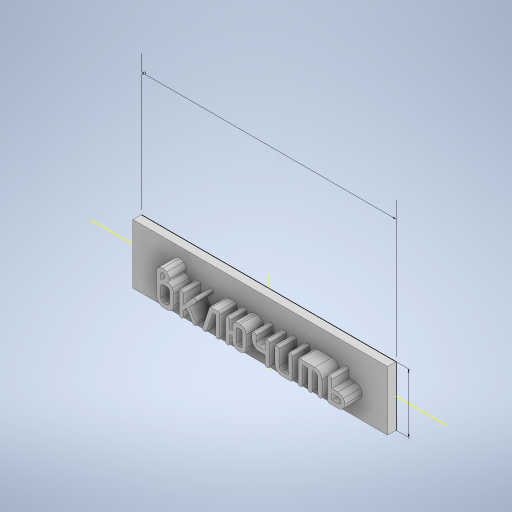
# Autodesk Inventor part: test hard text
Saved by Autodesk Inventor 2023.1 (Build 271208000, 208)
## iProperties
Created: 2023-03-05
Part Number: test hard text
Material: Типовые
Document SubType Name: Modeling
Designer: User
Density: 1 g/cm^3
Appearance: По умолчанию
Author: User
Autodesk Inventor part; units mm, degrees
ref_plane "YZ Plane" through (0, 0, 0) normal (1, 0, 0) x (0, 1, 0)
ref_plane "XZ Plane" through (0, 0, 0) normal (0, 1, 0) x (-1, 0, 0)
ref_plane "XY Plane" through (0, 0, 0) normal (0, 0, 1) x (1, 0, 0)
sketch "Эскиз1" plane through (0, 0, 0) normal (0, 0, 1) x (1, 0, 0)
  line L0 (-15, 3.5) -> (15, 3.5)
  line L1 (15, 3.5) -> (15, -3.5)
  line L2 (15, -3.5) -> (-15, -3.5)
  line L3 (-15, -3.5) -> (-15, 3.5)
  line L4 (0, -4.9) -> (0, 4.9) projected
  line L5 (-21, 0) -> (21, 0) projected
  line L6 (-10.6132, 2.2995) -> (12.268, 2.2995) construction
  line L7 (12.268, 2.2995) -> (12.268, -1.6939) construction
  line L8 (12.268, -1.6939) -> (-10.6132, -1.6939) construction
  line L9 (-10.6132, -1.6939) -> (-10.6132, 2.2995) construction
  spline S0 degree 2 poles (-8.9465, 1.1246) (-8.6066, 1.1246) (-8.3624, 0.8441) knots 0 0 0 1 1 1
  spline S1 degree 2 poles (-8.3624, 0.8441) (-8.1743, 0.6626) (-8.1743, 0.3061) knots 0 0 0 1 1 1
  line L10 (-8.1743, 0.3061) -> (-8.1743, -0.8556)
  spline S2 degree 2 poles (-8.1743, -0.8556) (-8.1743, -1.1988) (-8.6594, -1.6873) (-9.0059, -1.6873) knots 0 0 0 1 2 2 2
  line L11 (-9.0059, -1.6873) -> (-9.3954, -1.6873)
  spline S3 degree 2 poles (-9.3954, -1.6873) (-9.7353, -1.6873) (-10.2238, -1.2021) (-10.2238, -0.8556) knots 0 0 0 1 2 2 2
  line L12 (-10.2238, -0.8556) -> (-10.2238, 1.5471)
  spline S4 degree 2 poles (-10.2238, 1.5471) (-10.2238, 1.9002) (-9.9894, 2.1114) knots 0 0 0 1 1 1
  spline S5 degree 2 poles (-9.9894, 2.1114) (-9.7749, 2.2995) (-9.468, 2.2995) knots 0 0 0 1 1 1
  spline S6 degree 2 poles (-9.468, 2.2995) (-9.1611, 2.2995) (-9.0191, 2.1279) knots 0 0 0 1 1 1
  spline S7 degree 2 poles (-9.0191, 2.1279) (-8.7155, 1.9035) (-8.7155, 1.5504) knots 0 0 0 1 1 1
  spline S8 degree 2 poles (-8.7155, 1.5504) (-8.7155, 1.1939) (-8.9465, 1.1246) knots 0 0 0 1 1 1
  line L13 (-8.6759, -0.8589) -> (-8.6759, 0.3061)
  spline S9 degree 2 poles (-8.6759, 0.3061) (-8.6759, 0.4381) (-8.8739, 0.6362) (-9.0059, 0.6362) knots 0 0 0 1 2 2 2
  line L14 (-9.0059, 0.6362) -> (-9.3954, 0.6362)
  spline S10 degree 2 poles (-9.3954, 0.6362) (-9.5274, 0.6362) (-9.7221, 0.4414) (-9.7221, 0.3061) knots 0 0 0 1 2 2 2
  line L15 (-9.7221, 0.3061) -> (-9.7221, -0.8589)
  spline S11 degree 2 poles (-9.7221, -0.8589) (-9.7221, -0.9942) (-9.5274, -1.1889) (-9.3954, -1.1889) knots 0 0 0 1 2 2 2
  line L16 (-9.3954, -1.1889) -> (-9.0059, -1.1889)
  spline S12 degree 2 poles (-9.0059, -1.1889) (-8.8706, -1.1889) (-8.6759, -0.9942) (-8.6759, -0.8589) knots 0 0 0 1 2 2 2
  spline S13 degree 2 poles (-9.7221, 1.0025) (-9.6627, 1.0883) (-9.435, 1.2533) knots 0 0 0 1 1 1
  spline S14 degree 2 poles (-9.435, 1.2533) (-9.2172, 1.4249) (-9.2172, 1.5438) knots 0 0 0 1 1 1
  spline S15 degree 2 poles (-9.2172, 1.5438) (-9.2172, 1.6659) (-9.3063, 1.7451) knots 0 0 0 1 1 1
  spline S16 degree 2 poles (-9.3063, 1.7451) (-9.369, 1.7946) (-9.4713, 1.7946) knots 0 0 0 1 1 1
  spline S17 degree 2 poles (-9.4713, 1.7946) (-9.5769, 1.7946) (-9.6264, 1.7781) knots 0 0 0 1 1 1
  spline S18 degree 2 poles (-9.6264, 1.7781) (-9.7221, 1.6659) (-9.7221, 1.5438) knots 0 0 0 1 1 1
  line L17 (-9.7221, 1.5438) -> (-9.7221, 1.0025)
  spline S19 degree 2 poles (-6.6825, -0.4199) (-6.732, -0.4595) (-7.0489, -0.8391) knots 0 0 0 1 1 1
  line L18 (-7.0489, -0.8391) -> (-7.0489, -1.4364)
  spline S20 degree 2 poles (-7.0489, -1.4364) (-7.0489, -1.6873) (-7.2997, -1.6873) knots 0 0 0 1 1 1
  spline S21 degree 2 poles (-7.2997, -1.6873) (-7.5505, -1.6873) (-7.5505, -1.4364) knots 0 0 0 1 1 1
  line L19 (-7.5505, -1.4364) -> (-7.5505, 0.887)
  spline S22 degree 2 poles (-7.5505, 0.887) (-7.5505, 1.1378) (-7.2997, 1.1378) knots 0 0 0 1 1 1
  spline S23 degree 2 poles (-7.2997, 1.1378) (-7.0489, 1.1378) (-7.0489, 0.887) knots 0 0 0 1 1 1
  line L20 (-7.0489, 0.887) -> (-7.0489, -0.1988)
  line L21 (-7.0489, -0.1988) -> (-5.8805, 1.0883)
  spline S24 degree 2 poles (-5.8805, 1.0883) (-5.8508, 1.1477) (-5.7551, 1.1477) knots 0 0 0 1 1 1
  spline S25 degree 2 poles (-5.7551, 1.1477) (-5.6528, 1.1477) (-5.5043, 0.9827) (-5.5043, 0.8837) knots 0 0 0 1 2 2 2
  spline S26 degree 2 poles (-5.5043, 0.8837) (-5.5043, 0.7781) (-5.5802, 0.7022) knots 0 0 0 1 1 1
  line L22 (-5.5802, 0.7022) -> (-6.3426, -0.0833)
  line L23 (-6.3426, -0.0833) -> (-5.5604, -1.2747)
  spline S27 degree 2 poles (-5.5604, -1.2747) (-5.5043, -1.3605) (-5.5043, -1.4397) knots 0 0 0 1 1 1
  spline S28 degree 2 poles (-5.5043, -1.4397) (-5.5043, -1.5454) (-5.6627, -1.6939) (-5.7584, -1.6939) knots 0 0 0 1 2 2 2
  spline S29 degree 2 poles (-5.7584, -1.6939) (-5.8805, -1.6939) (-5.9168, -1.618) knots 0 0 0 1 1 1
  line L24 (-5.9168, -1.618) -> (-6.6825, -0.4199)
  spline S30 degree 2 poles (-2.7452, -1.4364) (-2.7452, -1.6873) (-2.996, -1.6873) knots 0 0 0 1 1 1
  spline S31 degree 2 poles (-2.996, -1.6873) (-3.2469, -1.6873) (-3.2469, -1.4364) knots 0 0 0 1 1 1
  line L25 (-3.2469, -1.4364) -> (-3.2469, 0.6395)
  line L26 (-3.2469, 0.6395) -> (-3.5934, 0.6395)
  line L27 (-3.5934, 0.6395) -> (-4.3195, -1.5553)
  spline S32 degree 2 poles (-4.3195, -1.5553) (-4.3591, -1.6873) (-4.534, -1.6873) knots 0 0 0 1 1 1
  spline S33 degree 2 poles (-4.534, -1.6873) (-4.7914, -1.6873) (-4.7914, -1.4463) knots 0 0 0 1 1 1
  spline S34 degree 2 poles (-4.7914, -1.4463) (-4.7914, -1.4001) (-4.7782, -1.3572) knots 0 0 0 1 1 1
  line L28 (-4.7782, -1.3572) -> (-3.996, 1.0058)
  spline S35 degree 2 poles (-3.996, 1.0058) (-3.9564, 1.1378) (-3.7749, 1.1378) knots 0 0 0 1 1 1
  line L29 (-3.7749, 1.1378) -> (-2.996, 1.1378)
  spline S36 degree 2 poles (-2.996, 1.1378) (-2.7452, 1.1378) (-2.7452, 0.887) knots 0 0 0 1 1 1
  line L30 (-2.7452, 0.887) -> (-2.7452, -1.4364)
  line L31 (-1.5769, -0.0272) -> (-1.3063, -0.0272)
  line L32 (-1.3063, -0.0272) -> (-1.3063, 0.4216)
  spline S37 degree 2 poles (-1.3063, 0.4216) (-1.3063, 0.7154) (-0.8904, 1.1378) (-0.5901, 1.1378) knots 0 0 0 1 2 2 2
  line L33 (-0.5901, 1.1378) -> (-0.3591, 1.1378)
  spline S38 degree 2 poles (-0.3591, 1.1378) (-0.0588, 1.1378) (0.3604, 0.7187) (0.3604, 0.4216) knots 0 0 0 1 2 2 2
  line L34 (0.3604, 0.4216) -> (0.3604, -0.9711)
  spline S39 degree 2 poles (0.3604, -0.9711) (0.3604, -1.2714) (-0.0555, -1.6873) (-0.3591, -1.6873) knots 0 0 0 1 2 2 2
  line L35 (-0.3591, -1.6873) -> (-0.5901, -1.6873)
  spline S40 degree 2 poles (-0.5901, -1.6873) (-0.8904, -1.6873) (-1.3063, -1.2714) (-1.3063, -0.9744) knots 0 0 0 1 2 2 2
  line L36 (-1.3063, -0.9744) -> (-1.3063, -0.5256)
  line L37 (-1.3063, -0.5256) -> (-1.5769, -0.5256)
  line L38 (-1.5769, -0.5256) -> (-1.5769, -1.4364)
  spline S41 degree 2 poles (-1.5769, -1.4364) (-1.5769, -1.6873) (-1.8277, -1.6873) knots 0 0 0 1 1 1
  spline S42 degree 2 poles (-1.8277, -1.6873) (-2.0786, -1.6873) (-2.0786, -1.4364) knots 0 0 0 1 1 1
  line L39 (-2.0786, -1.4364) -> (-2.0786, 0.887)
  spline S43 degree 2 poles (-2.0786, 0.887) (-2.0786, 1.1378) (-1.8277, 1.1378) knots 0 0 0 1 1 1
  spline S44 degree 2 poles (-1.8277, 1.1378) (-1.5769, 1.1378) (-1.5769, 0.887) knots 0 0 0 1 1 1
  line L40 (-1.5769, 0.887) -> (-1.5769, -0.0272)
  line L41 (-0.1413, -0.9744) -> (-0.1413, 0.4249)
  spline S45 degree 2 poles (-0.1413, 0.4249) (-0.1413, 0.5107) (-0.27, 0.6395) (-0.3591, 0.6395) knots 0 0 0 1 2 2 2
  line L42 (-0.3591, 0.6395) -> (-0.5901, 0.6395)
  spline S46 degree 2 poles (-0.5901, 0.6395) (-0.6792, 0.6395) (-0.8046, 0.5107) (-0.8046, 0.4249) knots 0 0 0 1 2 2 2
  line L43 (-0.8046, 0.4249) -> (-0.8046, -0.9744)
  spline S47 degree 2 poles (-0.8046, -0.9744) (-0.8046, -1.0635) (-0.6792, -1.1889) (-0.5901, -1.1889) knots 0 0 0 1 2 2 2
  line L44 (-0.5901, -1.1889) -> (-0.3591, -1.1889)
  spline S48 degree 2 poles (-0.3591, -1.1889) (-0.27, -1.1889) (-0.1413, -1.0635) (-0.1413, -0.9744) knots 0 0 0 1 2 2 2
  line L45 (2.5749, -0.0272) -> (2.5749, 0.887)
  spline S49 degree 2 poles (2.5749, 0.887) (2.5749, 1.1378) (2.8257, 1.1378) knots 0 0 0 1 1 1
  spline S50 degree 2 poles (2.8257, 1.1378) (3.0766, 1.1378) (3.0766, 0.887) knots 0 0 0 1 1 1
  line L46 (3.0766, 0.887) -> (3.0766, -1.4364)
  spline S51 degree 2 poles (3.0766, -1.4364) (3.0766, -1.6873) (2.8257, -1.6873) knots 0 0 0 1 1 1
  spline S52 degree 2 poles (2.8257, -1.6873) (2.5749, -1.6873) (2.5749, -1.4364) knots 0 0 0 1 1 1
  line L47 (2.5749, -1.4364) -> (2.5749, -0.5256)
  line L48 (2.5749, -0.5256) -> (1.8554, -0.5256)
  spline S53 degree 2 poles (1.8554, -0.5256) (1.5122, -0.5256) (1.0205, -0.0404) (1.0205, 0.3061) knots 0 0 0 1 2 2 2
  line L49 (1.0205, 0.3061) -> (1.0205, 0.887)
  spline S54 degree 2 poles (1.0205, 0.887) (1.0205, 1.1378) (1.2713, 1.1378) knots 0 0 0 1 1 1
  spline S55 degree 2 poles (1.2713, 1.1378) (1.5221, 1.1378) (1.5221, 0.887) knots 0 0 0 1 1 1
  line L50 (1.5221, 0.887) -> (1.5221, 0.3061)
  spline S56 degree 2 poles (1.5221, 0.3061) (1.5221, 0.1675) (1.7168, -0.0272) (1.8521, -0.0272) knots 0 0 0 1 2 2 2
  line L51 (1.8521, -0.0272) -> (2.5749, -0.0272)
  spline S57 degree 2 poles (5.7927, -1.4364) (5.7927, -1.6873) (5.5386, -1.6873) knots 0 0 0 1 1 1
  line L52 (5.5386, -1.6873) -> (4.5683, -1.6873)
  spline S58 degree 2 poles (4.5683, -1.6873) (4.2251, -1.6873) (3.7366, -1.2021) (3.7366, -0.8556) knots 0 0 0 1 2 2 2
  line L53 (3.7366, -0.8556) -> (3.7366, 0.887)
  spline S59 degree 2 poles (3.7366, 0.887) (3.7366, 1.1378) (3.9875, 1.1378) knots 0 0 0 1 1 1
  spline S60 degree 2 poles (3.9875, 1.1378) (4.2383, 1.1378) (4.2383, 0.887) knots 0 0 0 1 1 1
  line L54 (4.2383, 0.887) -> (4.2383, -0.8556)
  spline S61 degree 2 poles (4.2383, -0.8556) (4.2383, -0.9942) (4.433, -1.1889) (4.5683, -1.1889) knots 0 0 0 1 2 2 2
  line L55 (4.5683, -1.1889) -> (5.2911, -1.1889)
  line L56 (5.2911, -1.1889) -> (5.2911, 0.887)
  spline S62 degree 2 poles (5.2911, 0.887) (5.2911, 1.1378) (5.5419, 1.1378) knots 0 0 0 1 1 1
  spline S63 degree 2 poles (5.5419, 1.1378) (5.7927, 1.1378) (5.7927, 0.887) knots 0 0 0 1 1 1
  line L57 (5.7927, 0.887) -> (5.7927, -1.4364)
  line L58 (7.6145, 0.6395) -> (6.9544, 0.6395)
  line L59 (6.9544, 0.6395) -> (6.9544, -1.4364)
  spline S64 degree 2 poles (6.9544, -1.4364) (6.9544, -1.6873) (6.7036, -1.6873) knots 0 0 0 1 1 1
  spline S65 degree 2 poles (6.7036, -1.6873) (6.4528, -1.6873) (6.4528, -1.4364) knots 0 0 0 1 1 1
  line L60 (6.4528, -1.4364) -> (6.4528, 0.887)
  spline S66 degree 2 poles (6.4528, 0.887) (6.4528, 1.1378) (6.7036, 1.1378) knots 0 0 0 1 1 1
  line L61 (6.7036, 1.1378) -> (8.4429, 1.1378)
  spline S67 degree 2 poles (8.4429, 1.1378) (8.7894, 1.1378) (9.2779, 0.6494) (9.2779, 0.3061) knots 0 0 0 1 2 2 2
  line L62 (9.2779, 0.3061) -> (9.2779, -1.4364)
  spline S68 degree 2 poles (9.2779, -1.4364) (9.2779, -1.6873) (9.0271, -1.6873) knots 0 0 0 1 1 1
  spline S69 degree 2 poles (9.0271, -1.6873) (8.7762, -1.6873) (8.7762, -1.4364) knots 0 0 0 1 1 1
  line L63 (8.7762, -1.4364) -> (8.7762, 0.3094)
  spline S70 degree 2 poles (8.7762, 0.3094) (8.7762, 0.4414) (8.5782, 0.6395) (8.4462, 0.6395) knots 0 0 0 1 2 2 2
  line L64 (8.4462, 0.6395) -> (8.1162, 0.6395)
  line L65 (8.1162, 0.6395) -> (8.1162, -1.4364)
  spline S71 degree 2 poles (8.1162, -1.4364) (8.1162, -1.6873) (7.8653, -1.6873) knots 0 0 0 1 1 1
  spline S72 degree 2 poles (7.8653, -1.6873) (7.6145, -1.6873) (7.6145, -1.4364) knots 0 0 0 1 1 1
  line L66 (7.6145, -1.4364) -> (7.6145, 0.6395)
  line L67 (10.4396, -0.0272) -> (11.1591, -0.0272)
  spline S73 degree 2 poles (11.1591, -0.0272) (11.5551, -0.0272) (11.7993, -0.3374) knots 0 0 0 1 1 1
  spline S74 degree 2 poles (11.7993, -0.3374) (11.9941, -0.5256) (11.9941, -0.8556) knots 0 0 0 1 1 1
  spline S75 degree 2 poles (11.9941, -0.8556) (11.9941, -1.1922) (11.7993, -1.3374) knots 0 0 0 1 1 1
  spline S76 degree 2 poles (11.7993, -1.3374) (11.5551, -1.6873) (11.1591, -1.6873) knots 0 0 0 1 1 1
  line L68 (11.1591, -1.6873) -> (10.1888, -1.6873)
  spline S77 degree 2 poles (10.1888, -1.6873) (9.9379, -1.6873) (9.9379, -1.4364) knots 0 0 0 1 1 1
  line L69 (9.9379, -1.4364) -> (9.9379, 0.887)
  spline S78 degree 2 poles (9.9379, 0.887) (9.9379, 1.1378) (10.1888, 1.1378) knots 0 0 0 1 1 1
  spline S79 degree 2 poles (10.1888, 1.1378) (10.4396, 1.1378) (10.4396, 0.887) knots 0 0 0 1 1 1
  line L70 (10.4396, 0.887) -> (10.4396, -0.0272)
  line L71 (10.4396, -0.5256) -> (10.4396, -1.1889)
  line L72 (10.4396, -1.1889) -> (11.1591, -1.1889)
  spline S80 degree 2 poles (11.1591, -1.1889) (11.3175, -1.1889) (11.4726, -1.0701) knots 0 0 0 1 1 1
  spline S81 degree 2 poles (11.4726, -1.0701) (11.4924, -0.9942) (11.4924, -0.8556) knots 0 0 0 1 1 1
  spline S82 degree 2 poles (11.4924, -0.8556) (11.4924, -0.7203) (11.4759, -0.6444) knots 0 0 0 1 1 1
  spline S83 degree 2 poles (11.4759, -0.6444) (11.3175, -0.5256) (11.1591, -0.5256) knots 0 0 0 1 1 1
  line L73 (11.1591, -0.5256) -> (10.4396, -0.5256)
  point P0 (0, 0)
  dimension "d0" = 7
  dimension "d1" = 30
  constraints: 8 end point, 2 parallel, 1 horizontal, 1 perpendicular, 4 other
  measures "d0" distance between parallel lines of L2 L0
  measures "d1" distance between parallel lines of L3 L1
extrude "Выдавливание1" add sketch "Эскиз1" along normal blind 1 contours L0 L4 S38 L33 S37 L32 L5 L40 S44 S43 L39 L30 S36 L29 S35 L28 L22 S26 S25 S24 L21 L20 S23 S22 L19 L10 S1 S0 S8 S7 S6 S5 S4 L12 L3 | L0 L1 L5 L70 S79 S78 L69 L62 S67 L61 S66 L60 L57 S63 S62 L56 L54 S60 S59 L53 L46 S50 S49 L45 S56 L50 S55 S54 L49 S53 L34 S38 L4 | L5 L12 S3 L11 S2 L10 L19 S21 S20 L18 S19 L24 S29 S28 S27 L23 L22 L28 S34 S33 S32 L27 L25 S31 S30 L30 L39 S42 S41 L38 L37 L36 S40 L35 S39 L4 L2 L3 | S38 L34 L5 L4 | L4 L5 L41 S45 L42 S46 L43 L32 S37 L33 S38 | L12 S4 S5 S6 S7 S8 S0 S1 L10 L5 L13 S9 L14 S10 L15 | L5 L15 S11 L16 S12 L13 L10 S2 L11 S3 L12 | L1 L2 L4 S39 L34 L5 S53 L48 L47 S52 S51 L46 L53 S58 L52 S57 L57 L60 S65 S64 L59 L66 S72 S71 L65 L63 S69 S68 L62 L69 S77 L68 S76 S75 S74 S73 L67 L70 | L5 L34 S39 L4 | L4 S39 L35 S40 L36 L37 L38 S41 S42 L39 L5 L40 L31 L32 L43 S47 L44 S48 L41 | L15 S10 L14 S9 L13 L5 | L5 L13 S12 L16 S11 L15 | L70 L67 S73 S74 S75 S76 L68 S77 L69 L5 | L5 L69 S78 S79 L70 | L41 S48 L44 S47 L43 L5 | L5 L43 S46 L42 S45 L41 | S53 L49 S54 S55 L50 S56 L5 | L5 S56 L51 L45 L46 S51 S52 L47 L48 S53 | L62 S68 S69 L63 L5 | L5 L63 S70 L64 L65 L66 L58 L59 L60 S66 L61 S67 L62 | L32 L31 L40 L5 | L5 L45 L51 S56 | L19 S22 S23 L20 L5 | L5 L20 L21 L22 L23 S27 S28 S29 L24 S19 L18 S20 S21 L19 | L5 L65 L64 S70 L63 | L5 L39 S43 S44 L40 | L45 S49 S50 L46 L5 | L5 L21 L20 | L65 S71 S72 L66 L5 | L21 S24 S25 S26 L22 L5 | L5 L59 L58 L66 | L30 S30 S31 L25 L5 | L5 L25 L26 L27 L28 S35 L29 S36 L30 | L53 S59 S60 L54 L5 | L5 L54 S61 L55 L56 L57 S57 L52 S58 L53 | L59 S64 S65 L60 L5 | L5 L27 L26 L25 | L5 L56 L55 S61 L54 | L5 L27 S32 S33 S34 L28 | L56 S62 S63 L57 L5 | L17 S18 S17 S16 S15 S14 S13 | L73 S83 S82 S81 S80 L72 L71
extrude "Выдавливание2" add sketch "Эскиз1" along normal blind 3 contours S38 L34 L5 L4 | L4 L5 L41 S45 L42 S46 L43 L32 S37 L33 S38 | L12 S4 S5 S6 S7 S8 S0 S1 L10 L5 L13 S9 L14 S10 L15 | L5 L15 S11 L16 S12 L13 L10 S2 L11 S3 L12 | L5 L34 S39 L4 | L4 S39 L35 S40 L36 L37 L38 S41 S42 L39 L5 L40 L31 L32 L43 S47 L44 S48 L41 | L70 L67 S73 S74 S75 S76 L68 S77 L69 L5 | L5 L69 S78 S79 L70 | S53 L49 S54 S55 L50 S56 L5 | L5 S56 L51 L45 L46 S51 S52 L47 L48 S53 | L62 S68 S69 L63 L5 | L5 L63 S70 L64 L65 L66 L58 L59 L60 S66 L61 S67 L62 | L19 S22 S23 L20 L5 | L5 L20 L21 L22 L23 S27 S28 S29 L24 S19 L18 S20 S21 L19 | L5 L39 S43 S44 L40 | L45 S49 S50 L46 L5 | L65 S71 S72 L66 L5 | L21 S24 S25 S26 L22 L5 | L30 S30 S31 L25 L5 | L5 L25 L26 L27 L28 S35 L29 S36 L30 | L53 S59 S60 L54 L5 | L5 L54 S61 L55 L56 L57 S57 L52 S58 L53 | L59 S64 S65 L60 L5 | L5 L27 S32 S33 S34 L28 | L56 S62 S63 L57 L5
